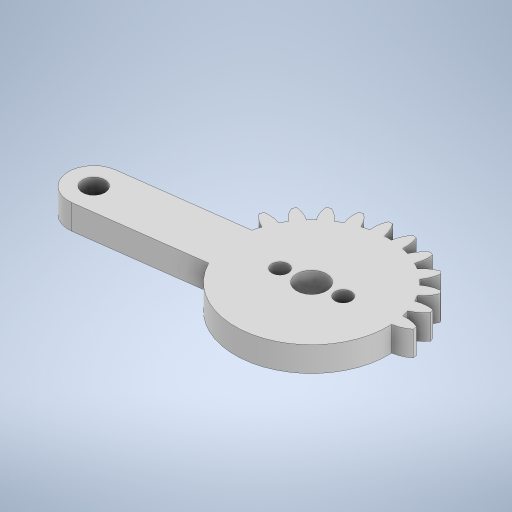
# Autodesk Inventor part: gear2
Saved by Autodesk Inventor 2024.1 (Build 281209000, 209)
## iProperties
Created: 2023-12-01
Part Number: gear2
Material: Generic
Document SubType Name: Modeling
Designer: vilas
Density: 1 g/cm^3
Appearance: Default
Author: vilas
Autodesk Inventor part; units mm, degrees
ref_plane "YZ Plane" through (0, 0, 0) normal (1, 0, 0) x (0, 1, 0)
ref_plane "XZ Plane" through (0, 0, 0) normal (0, 1, 0) x (-1, 0, 0)
ref_plane "XY Plane" through (0, 0, 0) normal (0, 0, 1) x (1, 0, 0)
sketch "Sketch1" plane through (0, 0, 0) normal (0, 1, 0) x (-1, 0, 0)
  arc A0 (-88.2418, 370.4906) -> (-114.8998, 572.0282) centre (-101.9147, 471.2139) ccw
  line L0 (-88.2418, 370.4906) -> (-573.2931, 306.6646)
  line L1 (-114.8998, 572.0282) -> (-600.8636, 508.0822)
  circle A1 centre (-101.9147, 471.2139) radius 45
  circle A2 centre (-874.6108, 368.0153) radius 60
  line L2 (-101.9147, 471.2139) -> (-874.6108, 368.0153) construction
  line L3 (-874.6108, 368.0153) -> (-1133.932, 333.3813) construction
  line L4 (-762.6053, 382.9744) -> (-756.3631, 336.2359) construction
  circle A3 centre (-762.6053, 382.9744) radius 33
  line L5 (-986.6163, 353.0563) -> (-993.4793, 404.4435) construction
  circle A4 centre (-986.6163, 353.0563) radius 33
  arc A5 (-529.8849, 234.3477) -> (-581.3863, 275.4105) centre (-630.6569, 160.7865) ccw
  arc A6 (-601.2954, 227.1078) -> (-536.0207, 219.8384) centre (-554.2466, 352.8807) ccw
  line L6 (-536.0207, 219.8384) -> (-529.8849, 234.3477)
  arc A7 (-647.0779, 161.1698) -> (-585.9089, 137.2539) centre (-569.0799, 270.48) ccw
  arc A8 (-576.2269, 149.6807) -> (-615.3456, 202.6738) centre (-692.6042, 104.7077) ccw
  line L7 (-585.9089, 137.2539) -> (-576.2269, 149.6807)
  arc A9 (-708.3665, 109.3281) -> (-655.4716, 70.3954) centre (-604.7346, 194.7263) ccw
  arc A10 (-642.9032, 79.8928) -> (-666.9734, 141.2049) centre (-766.955, 66.5729) ccw
  line L8 (-655.4716, 70.3954) -> (-642.9032, 79.8928)
  arc A11 (-780.9843, 75.1155) -> (-739.9683, 23.8191) centre (-658.7809, 130.7818) ccw
  arc A12 (-725.3701, 29.74) -> (-732.7513, 95.1928) centre (-848.6423, 48.981) ccw
  line L9 (-739.9683, 23.8191) -> (-725.3701, 29.74)
  arc A13 (-859.9826, 60.8635) -> (-833.6407, 0.6993) centre (-727.5357, 83.0045) ccw
  arc A14 (-818.0074, 2.6401) -> (-808.1967, 67.7731) centre (-932.0993, 53.1307) ccw
  line L10 (-833.6407, 0.6993) -> (-818.0074, 2.6401)
  arc A15 (-939.9778, 67.5434) -> (-930.1051, 2.6114) centre (-806.3134, 54.6501) ccw
  arc A16 (-914.5022, 0.4399) -> (-888.1681, 60.8143) centre (-1011.6386, 78.7392) ccw
  line L11 (-930.1051, 2.6114) -> (-914.5022, 0.4399)
  arc A17 (-1015.5184, 94.6999) -> (-1022.7877, 29.4253) centre (-889.7454, 47.6511) ccw
  arc A18 (-1008.2784, 23.2894) -> (-967.2157, 74.7909) centre (-1081.8397, 124.0615) ccw
  line L12 (-1022.7877, 29.4253) -> (-1008.2784, 23.2894)
  arc A19 (-1081.4563, 140.4825) -> (-1105.3722, 79.3134) centre (-972.1461, 62.4844) ccw
  arc A20 (-1092.9455, 69.6314) -> (-1039.9523, 108.7502) centre (-1137.9184, 186.0088) ccw
  line L13 (-1105.3722, 79.3134) -> (-1092.9455, 69.6314)
  arc A21 (-1133.298, 201.771) -> (-1172.2308, 148.8762) centre (-1047.8999, 98.1391) ccw
  arc A22 (-1162.7333, 136.3078) -> (-1101.4212, 160.3779) centre (-1176.0532, 260.3595) ccw
  line L14 (-1172.2308, 148.8762) -> (-1162.7333, 136.3078)
  arc A23 (-1167.5107, 274.3889) -> (-1218.807, 233.3729) centre (-1111.8443, 152.1854) ccw
  arc A24 (-1212.8861, 218.7746) -> (-1147.4333, 226.1559) centre (-1193.6451, 342.0469) ccw
  line L15 (-1218.807, 233.3729) -> (-1212.8861, 218.7746)
  arc A25 (-1181.7626, 353.3872) -> (-1241.9268, 327.0452) centre (-1159.6216, 220.9402) ccw
  arc A26 (-1239.986, 311.412) -> (-1174.8531, 301.6013) centre (-1189.4955, 425.5039) ccw
  line L16 (-1241.9268, 327.0452) -> (-1239.986, 311.412)
  arc A27 (-581.3863, 275.4105) -> (-573.2931, 306.6646) centre (-874.6108, 368.0153) ccw
  arc A28 (-615.3456, 202.6738) -> (-601.2954, 227.1078) centre (-874.6108, 368.0153) ccw
  arc A29 (-666.9734, 141.2049) -> (-647.0779, 161.1698) centre (-874.6108, 368.0153) ccw
  arc A30 (-732.7513, 95.1928) -> (-708.3665, 109.3281) centre (-874.6108, 368.0153) ccw
  arc A31 (-808.1967, 67.7731) -> (-780.9843, 75.1155) centre (-874.6108, 368.0153) ccw
  arc A32 (-888.1681, 60.8143) -> (-859.9826, 60.8635) centre (-874.6108, 368.0153) ccw
  arc A33 (-967.2157, 74.7909) -> (-939.9778, 67.5434) centre (-874.6108, 368.0153) ccw
  arc A34 (-1039.9523, 108.7502) -> (-1015.5184, 94.6999) centre (-874.6108, 368.0153) ccw
  arc A35 (-1101.4212, 160.3779) -> (-1081.4563, 140.4825) centre (-874.6108, 368.0153) ccw
  arc A36 (-1147.4333, 226.1559) -> (-1133.298, 201.771) centre (-874.6108, 368.0153) ccw
  arc A37 (-600.8636, 508.0822) -> (-1181.7626, 353.3872) centre (-874.6108, 368.0153) ccw
  arc A38 (-1174.8531, 301.6013) -> (-1167.5107, 274.3889) centre (-874.6108, 368.0153) ccw
  point P0 (0, 0)
  dimension "d1" = 90
  dimension "d3" = 120
  dimension "d6" = 113
  dimension "d7" = 66
  dimension "d8" = 113
  dimension "d9" = 66
  dimension "d12" = 150
  constraints: 70 point on circle, 39 centre point, 34 end point, 4 coincident, 2 perpendicular, 2 point on line, 1 collinear, 91 other
  measures "d1" diameter of A1
  measures "d3" diameter of A2
  measures "d6" distance from line of L4 A27.centre
  measures "d7" diameter of A3
  measures "d8" distance from line of L5 A27.centre
  measures "d9" diameter of A4
extrude "Extrusion1" add sketch "Sketch1" along normal blind 100
scale "Scale1" factors (0.1, 0.1, 0.1) then translate (686.3448, 0, 344.677) bodies 1
body "Solid1"
